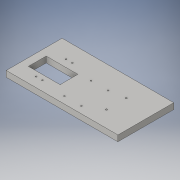
# Autodesk Inventor part: RectangleFifteen1
Saved by Autodesk Inventor 2016 (Build 200138000, 138)
## iProperties
Created: 2017-04-26
Part Number: RectangleFifteen1
Material: Generic
Document SubType Name: Modeling
Designer: Evan Phil George
Density: 1 g/cm^3
Appearance: Default
Author: Evan Phil George
Autodesk Inventor part; units mm, degrees
ref_plane "YZ Plane" through (0, 0, 0) normal (1, 0, 0) x (0, 1, 0)
ref_plane "XZ Plane" through (0, 0, 0) normal (0, 1, 0) x (-1, 0, 0)
ref_plane "XY Plane" through (0, 0, 0) normal (0, 0, 1) x (1, 0, 0)
sketch "Sketch1" plane through (0, 0, 0) normal (0, 1, 0) x (-1, 0, 0)
  line L0 (141, -70.5) -> (-141, -70.5)
  line L1 (-141, -70.5) -> (-141, 70.5)
  line L2 (-141, 70.5) -> (141, 70.5)
  line L3 (141, 70.5) -> (141, -70.5)
  line L4 (141, -70.5) -> (-141, 70.5) construction
  line L5 (-141, -70.5) -> (141, 70.5) construction
  point P0 (0, 0)
  dimension "d0" = 282
  dimension "d1" = 141
  constraints: 12 end point, 2 midpoint, 2 parallel, 1 horizontal, 1 perpendicular
  measures "d0" distance of L1.end L2.end
  measures "d1" distance of L0.end L1.end
extrude "RectangleFace" add sketch "Sketch1" along normal blind 15
sketch "Sketch2" plane through (0, 15, 0) normal (0, 1, 0) x (1, 0, 0)
  line L0 (141, 70.5) -> (-141, 70.5) projected
  line L1 (0, 70.5) -> (0, -11.1)
  line L2 (0, -11.1) -> (-82, -11.1)
  line L3 (-122, 11.4) -> (-42, 11.4)
  line L4 (-42, 11.4) -> (-42, -33.6)
  line L5 (-42, -33.6) -> (-122, -33.6)
  line L6 (-122, -33.6) -> (-122, 11.4)
  line L7 (-122, 11.4) -> (-42, -33.6) construction
  line L8 (-42, 11.4) -> (-122, -33.6) construction
  point P0 (0, 0)
  dimension "d4" = 81.6
  dimension "d5" = 82
  dimension "d6" = 80
  dimension "d7" = 45
  constraints: 16 end point, 3 midpoint, 2 parallel, 2 perpendicular, 1 horizontal, 1 vertical
  measures "d4" distance of L1.start L1.end
  measures "d5" distance of L1.end L2.end
  measures "d6" distance of L4.end L5.end
  measures "d7" distance of L3.end L4.end
extrude "RectangularCut" cut sketch "Sketch2" against normal blind 15
sketch "Sketch3" plane through (0, 15, 0) normal (0, 1, 0) x (1, 0, 0)
  line L0 (-42, 11.4) -> (-122, 11.4) projected
  line L1 (-82, 11.4) -> (-82, 29.4)
  line L2 (-122, -33.6) -> (-42, -33.6) projected
  line L3 (-82, -33.6) -> (-82, -46.1)
  line L4 (-82, 29.4) -> (-74, 29.4)
  line L5 (-82, 29.4) -> (-90, 29.4)
  line L6 (-82, -46.1) -> (-74, -46.1)
  line L7 (-82, -46.1) -> (-90, -46.1)
  circle A0 centre (-74, -46.1) radius 1.75
  circle A1 centre (-90, -46.1) radius 1.75
  circle A2 centre (-74, 29.4) radius 1.75
  circle A3 centre (-90, 29.4) radius 1.75
  point P0 (0, 0)
  dimension "d10" = 18
  dimension "d11" = 12.5
  dimension "d12" = 8
  dimension "d13" = 8
  dimension "d14" = 8
  dimension "d15" = 8
  dimension "d16" = 3.5
  dimension "d17" = 3.5
  dimension "d18" = 3.5
  dimension "d19" = 3.5
  constraints: 12 end point, 4 centre point, 4 coincident, 4 horizontal, 2 midpoint, 2 vertical
  measures "d10" distance of L1.start L1.end
  measures "d11" distance of L3.start L3.end
  measures "d12" distance of L1.end L4.end
  measures "d13" distance of L1.end L5.end
  measures "d14" distance of L3.end L6.end
  measures "d15" distance of L3.end L7.end
  measures "d16" diameter of A0
  measures "d17" diameter of A1
  measures "d18" diameter of A2
  measures "d19" diameter of A3
extrude "AxleSupportHoles" cut sketch "Sketch3" against normal blind 15
sketch "Sketch4" plane through (0, 15, 0) normal (0, 1, 0) x (1, 0, 0)
  line L0 (141, 70.5) -> (-141, 70.5) projected
  line L1 (0, 70.5) -> (0, -19.5)
  line L2 (0, -19.5) -> (10, -19.5)
  line L3 (-15.5, 18.25) -> (35.5, 18.25)
  line L4 (35.5, 18.25) -> (35.5, -57.25)
  line L5 (35.5, -57.25) -> (-15.5, -57.25)
  line L6 (-15.5, -57.25) -> (-15.5, 18.25)
  line L7 (-15.5, 18.25) -> (35.5, -57.25) construction
  line L8 (35.5, 18.25) -> (-15.5, -57.25) construction
  line L9 (-15.5, 18.25) -> (-11.5, 18.25)
  line L10 (-11.5, 18.25) -> (-11.5, 14.25)
  line L11 (35.5, 18.25) -> (31.5, 18.25)
  line L12 (31.5, 18.25) -> (31.5, 14.25)
  line L13 (-15.5, -57.25) -> (-11.5, -57.25)
  line L14 (-11.5, -57.25) -> (-11.5, -53.25)
  line L15 (35.5, -57.25) -> (31.5, -57.25)
  line L16 (31.5, -57.25) -> (31.5, -53.25)
  circle A0 centre (-11.5, -53.25) radius 1.75
  circle A1 centre (31.5, -53.25) radius 1.75
  circle A2 centre (31.5, 14.25) radius 1.75
  circle A3 centre (-11.5, 14.25) radius 1.75
  point P0 (0, 0)
  dimension "d22" = 90
  dimension "d23" = 10
  dimension "d24" = 51
  dimension "d25" = 75.5
  dimension "d26" = 4
  dimension "d27" = 4
  dimension "d28" = 4
  dimension "d29" = 4
  dimension "d30" = 4
  dimension "d31" = 4
  dimension "d32" = 4
  dimension "d33" = 4
  dimension "d34" = 3.5
  dimension "d35" = 3.5
  dimension "d36" = 3.5
  dimension "d37" = 3.5
  constraints: 32 end point, 6 perpendicular, 4 centre point, 4 coincident, 4 point on line, 3 midpoint, 2 parallel, 1 horizontal, 1 vertical
  measures "d22" distance of L1.start L1.end
  measures "d23" distance of L1.end L2.end
  measures "d24" distance of L4.end L5.end
  measures "d25" distance of L3.end L4.end
  measures "d26" distance of L3.start L9.end
  measures "d27" distance of L9.end L10.end
  measures "d28" distance of L3.end L11.end
  measures "d29" distance of L11.end L12.end
  measures "d30" distance of L5.end L13.end
  measures "d31" distance of L13.end L14.end
  measures "d32" distance of L4.end L15.end
  measures "d33" distance of L15.end L16.end
  measures "d34" diameter of A0
  measures "d35" diameter of A1
  measures "d36" diameter of A2
  measures "d37" diameter of A3
extrude "DriverHoles" cut sketch "Sketch4" against normal blind 15 contours A0 | A1 | A2 | A3
sketch "Sketch5" plane through (0, 15, 0) normal (0, 1, 0) x (1, 0, 0)
  line L0 (-141, 70.5) -> (141, 70.5) projected
  line L1 (141, 70.5) -> (71, 70.5)
  line L2 (71, 70.5) -> (71, 20.5)
  line L3 (71, 70.5) -> (121, 70.5) construction
  line L4 (71, 20.5) -> (71, -29.5)
  circle A0 centre (71, 20.5) radius 2
  circle A1 centre (71, -29.5) radius 2
  point P0 (0, 0)
  dimension "d40" = 70
  dimension "d41" = 50
  dimension "d42" = 90
  dimension "d43" = 50
  dimension "d44" = 180
  dimension "d45" = 4
  dimension "d46" = 4
  constraints: 8 end point, 2 centre point, 2 coincident, 2 perpendicular, 1 collinear, 1 horizontal, 1 point on line
  measures "d40" distance of L0.end L1.end
  measures "d41" distance of L1.end L2.end
  measures "d42" angle of L2 L3
  measures "d43" distance of L2.end L4.end
  measures "d44" angle of L4 L2
  measures "d45" diameter of A0
  measures "d46" diameter of A1
extrude "Extrusion5" cut sketch "Sketch5" against normal blind 15
body "Solid1"
